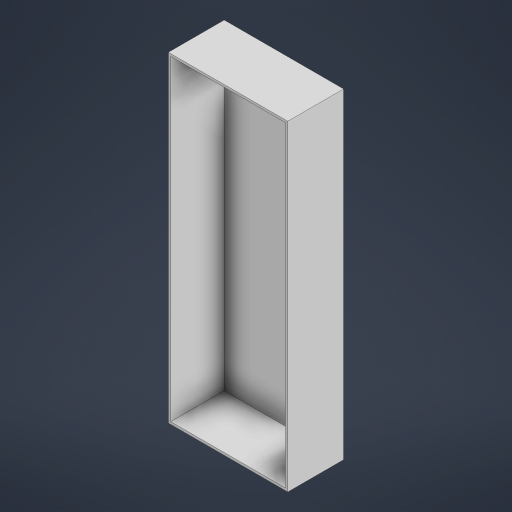
# Autodesk Inventor part: PAX
Saved by Autodesk Inventor 2024.2 (Build 282272000, 272)
## iProperties
Created: 2025-08-11
Part Number: PAX
Material: Generic
Document SubType Name: Modeling
Designer: Luca
Density: 1 g/cm^3
Appearance: Default
Author: Luca
Autodesk Inventor part; units mm, degrees
ref_plane "YZ Plane" through (0, 0, 0) normal (1, 0, 0) x (0, 1, 0)
ref_plane "XZ Plane" through (0, 0, 0) normal (0, 1, 0) x (-1, 0, 0)
ref_plane "XY Plane" through (0, 0, 0) normal (0, 0, 1) x (1, 0, 0)
sketch "Sketch1" plane through (0, 0, 0) normal (0, 1, 0) x (-1, 0, 0)
  line L0 (374, 0) -> (-374, 0)
  line L1 (-374, 0) -> (-374, 350)
  line L2 (-374, 350) -> (374, 350)
  line L3 (374, 350) -> (374, 0)
  point P0 (0, 0)
  point P1 (0, 0)
  dimension "d0" = 350
  dimension "d1" = 748
  constraints: 8 end point, 2 parallel, 1 coincident, 1 horizontal, 1 midpoint, 1 perpendicular
  measures "d0" distance of L0.end L1.end
  measures "d1" distance of L0.start L0.end
extrude "Extrusion1" add sketch "Sketch1" along normal blind 2012
shell "Shell1" thickness 15 removed faces 1 at (-124.6667, 670.6667, 350)
body "Solid1"
